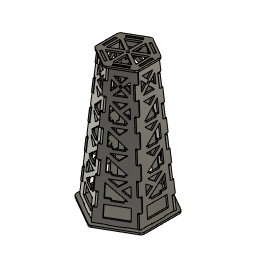
windmill v4 (Autodesk Fusion 360 design; units mm, degrees)
Autodesk Fusion 360 part; units mm, degrees
sketch "Sketch2" plane through (0, 0, 0) normal (0, 0, 1) x (1, 0, 0)
  line L0 (129.0294, -114.8559) -> (68.6327, -149.726)
  arc A0 (68.6327, -149.726) -> (63.1421, -149.726) centre (65.8874, -144.9709) cw
  line L1 (63.1421, -149.726) -> (2.7453, -114.8559)
  arc A1 (2.7453, -114.8559) -> (0, -110.1009) centre (5.4906, -110.1009) cw
  line L2 (0, -110.1009) -> (0, -40.3607)
  arc A2 (0, -40.3607) -> (2.7453, -35.6057) centre (5.4906, -40.3607) cw
  line L3 (2.7453, -35.6057) -> (63.1421, -0.7356)
  arc A3 (63.1421, -0.7356) -> (68.6327, -0.7356) centre (65.8874, -5.4906) cw
  line L4 (68.6327, -0.7356) -> (129.0294, -35.6057)
  arc A4 (129.0294, -35.6057) -> (131.7748, -40.3607) centre (126.2841, -40.3607) cw
  line L5 (131.7748, -40.3607) -> (131.7748, -110.1009)
  arc A5 (131.7748, -110.1009) -> (129.0294, -114.8559) centre (126.2841, -110.1009) cw
  line L6 (84.6564, -133.0999) -> (106.6189, -120.4198)
  line L7 (106.6189, -120.4198) -> (104.7697, -117.217)
  line L8 (104.7697, -117.217) -> (82.8073, -129.897)
  line L9 (82.8073, -129.897) -> (84.6564, -133.0999)
  line L10 (47.1183, -133.0997) -> (25.1558, -120.4197)
  line L11 (25.1558, -120.4197) -> (27.005, -117.2168)
  line L12 (27.005, -117.2168) -> (48.9674, -129.8969)
  line L13 (48.9674, -129.8969) -> (47.1183, -133.0997)
  line L14 (47.1183, -17.3616) -> (25.1558, -30.0416)
  line L15 (25.1558, -30.0416) -> (27.005, -33.2445)
  line L16 (27.005, -33.2445) -> (48.9674, -20.5645)
  line L17 (48.9674, -20.5645) -> (47.1183, -17.3616)
  line L18 (121.6896, -62.5506) -> (125.388, -62.5506)
  line L19 (125.388, -62.5506) -> (125.388, -87.9107)
  line L20 (125.388, -87.9107) -> (121.6896, -87.9107)
  line L21 (121.6896, -87.9107) -> (121.6896, -62.5506)
  line L22 (6.3867, -62.5506) -> (10.0851, -62.5506)
  line L23 (10.0851, -62.5506) -> (10.0851, -87.9107)
  line L24 (10.0851, -87.9107) -> (6.3867, -87.9107)
  line L25 (6.3867, -87.9107) -> (6.3867, -62.5506)
  line L26 (84.6564, -17.3616) -> (106.6189, -30.0416)
  line L27 (106.6189, -30.0416) -> (104.7697, -33.2445)
  line L28 (104.7697, -33.2445) -> (82.8073, -20.5645)
  line L29 (82.8073, -20.5645) -> (84.6564, -17.3616)
extrude "Extrude1" add sketch "Sketch2" along normal blind 3.175 makes body 1
sketch "Sketch4" plane through (0, 0, 0) normal (0, 0, 1) x (1, 0, 0)
  line L0 (18.968, -3.1158) -> (17.7262, -25.4072)
  line L1 (17.7262, -25.4072) -> (11.8611, -25.4072)
  arc A0 (11.3622, -25.8815) -> (11.8611, -25.4072) centre (11.8611, -25.9067) cw
  line L2 (11.3622, -25.8815) -> (10.145, -49.9595)
  arc A1 (10.6433, -50.4837) -> (10.145, -49.9595) centre (10.6433, -49.9847) cw
  line L3 (10.6433, -50.4837) -> (16.4585, -50.4837)
  line L4 (16.4585, -50.4837) -> (15.1903, -76.1274)
  line L5 (15.1903, -76.1274) -> (9.3252, -76.1274)
  arc A2 (8.8263, -76.6016) -> (9.3252, -76.1274) centre (9.3252, -76.6269) cw
  line L6 (8.8263, -76.6016) -> (7.6091, -100.6797)
  arc A3 (8.1074, -101.2038) -> (7.6091, -100.6797) centre (8.1074, -100.7049) cw
  line L7 (8.1074, -101.2038) -> (13.9226, -101.2038)
  line L8 (13.9226, -101.2038) -> (12.6544, -126.8475)
  line L9 (12.6544, -126.8475) -> (6.7893, -126.8475)
  arc A4 (6.2904, -127.3218) -> (6.7893, -126.8475) centre (6.7893, -127.347) cw
  line L10 (6.2904, -127.3218) -> (5.0727, -151.3998)
  arc A5 (5.571, -151.9239) -> (5.0727, -151.3998) centre (5.571, -151.425) cw
  line L11 (5.571, -151.9239) -> (11.3862, -151.9239)
  line L12 (11.3862, -151.9239) -> (10.1185, -177.5676)
  line L13 (10.1185, -177.5676) -> (4.2534, -177.5676)
  arc A6 (3.7545, -178.0419) -> (4.2534, -177.5676) centre (4.2534, -178.0671) cw
  line L14 (3.7545, -178.0419) -> (2.5368, -202.1199)
  arc A7 (3.0351, -202.644) -> (2.5368, -202.1199) centre (3.0351, -202.1451) cw
  line L15 (3.0351, -202.644) -> (8.8503, -202.644)
  line L16 (8.8503, -202.644) -> (7.5826, -228.2878)
  line L17 (7.5826, -228.2878) -> (1.7174, -228.2878)
  arc A8 (1.2188, -228.762) -> (1.7174, -228.2878) centre (1.7174, -228.787) cw
  line L18 (1.2188, -228.762) -> (0.0006, -253.0765)
  arc A9 (0.4992, -253.6006) -> (0.0006, -253.0765) centre (0.4992, -253.1015) cw
  line L19 (0.4992, -253.6006) -> (23.7494, -253.6006)
  line L20 (23.7494, -253.6006) -> (23.7494, -255.7351)
  arc A10 (24.2566, -256.2423) -> (23.7494, -255.7351) centre (24.2566, -255.7351) cw
  line L21 (24.2566, -256.2423) -> (48.6023, -256.2423)
  arc A11 (49.1095, -255.7351) -> (48.6023, -256.2423) centre (48.6023, -255.7351) cw
  line L22 (49.1095, -255.7351) -> (49.1095, -253.6006)
  line L23 (49.1095, -253.6006) -> (66.0203, -253.6006)
  arc A12 (66.5186, -253.077) -> (66.0203, -253.6006) centre (66.0203, -253.1017) cw
  line L24 (66.5186, -253.077) -> (65.2763, -228.0041)
  line L25 (65.2763, -228.0041) -> (71.0904, -228.0041)
  arc A13 (71.5898, -227.4788) -> (71.0904, -228.0041) centre (71.0904, -227.5041) cw
  line L26 (71.5898, -227.4788) -> (70.3726, -203.4009)
  arc A14 (69.8748, -202.9277) -> (70.3726, -203.4009) centre (69.8748, -203.4261) cw
  line L27 (69.8748, -202.9277) -> (64.0086, -202.9277)
  line L28 (64.0086, -202.9277) -> (62.7404, -177.284)
  line L29 (62.7404, -177.284) -> (68.5545, -177.284)
  arc A15 (69.0539, -176.7587) -> (68.5545, -177.284) centre (68.5545, -176.784) cw
  line L30 (69.0539, -176.7587) -> (67.8367, -152.6808)
  arc A16 (67.3389, -152.2076) -> (67.8367, -152.6808) centre (67.3389, -152.706) cw
  line L31 (67.3389, -152.2076) -> (61.4727, -152.2076)
  line L32 (61.4727, -152.2076) -> (60.2058, -126.5889)
  arc A17 (60.2058, -126.5889) -> (60.2296, -126.5639) centre (60.2296, -126.5878) cw
  line L33 (60.2296, -126.5639) -> (66.0186, -126.5639)
  arc A18 (66.518, -126.0386) -> (66.0186, -126.5639) centre (66.0186, -126.0639) cw
  line L34 (66.518, -126.0386) -> (65.3016, -101.9861)
  arc A19 (64.7771, -101.4875) -> (65.3016, -101.9861) centre (64.7771, -102.0126) cw
  line L35 (64.7771, -101.4875) -> (58.9363, -101.4875)
  line L36 (58.9363, -101.4875) -> (57.6686, -75.8438)
  line L37 (57.6686, -75.8438) -> (63.4827, -75.8438)
  arc A20 (63.9821, -75.3184) -> (63.4827, -75.8438) centre (63.4827, -75.3437) cw
  line L38 (63.9821, -75.3184) -> (62.7643, -51.2405)
  arc A21 (62.2666, -50.7673) -> (62.7643, -51.2405) centre (62.2666, -51.2657) cw
  line L39 (62.2666, -50.7673) -> (56.4004, -50.7673)
  line L40 (56.4004, -50.7673) -> (55.1327, -25.1236)
  line L41 (55.1327, -25.1236) -> (60.9474, -25.1236)
  arc A22 (61.4431, -24.5991) -> (60.9474, -25.1236) centre (60.9474, -24.627) cw
  line L42 (61.4431, -24.5991) -> (60.2312, -3.1153)
  arc A23 (59.7301, -2.6417) -> (60.2312, -3.1153) centre (59.7301, -3.1436) cw
  line L43 (59.7301, -2.6417) -> (49.1095, -2.6417)
  line L44 (49.1095, -2.6417) -> (49.1095, -0.5072)
  arc A24 (48.6023, 0) -> (49.1095, -0.5072) centre (48.6023, -0.5072) cw
  line L45 (48.6023, 0) -> (24.2566, 0)
  arc A25 (23.7494, -0.5072) -> (24.2566, 0) centre (24.2566, -0.5072) cw
  line L46 (23.7494, -0.5072) -> (23.7494, -2.6417)
  line L47 (23.7494, -2.6417) -> (19.4693, -2.6417)
  arc A26 (18.968, -3.1158) -> (19.4693, -2.6417) centre (19.4693, -3.1437) cw
  line L48 (21.7542, -63.9071) -> (20.9934, -88.2533)
  arc A27 (21.4847, -88.7602) -> (20.9934, -88.2533) centre (21.4847, -88.2686) cw
  line L49 (21.4847, -88.7602) -> (26.412, -88.7602)
  arc A28 (26.412, -88.7602) -> (26.9192, -89.2674) centre (26.412, -89.2674) cw
  line L50 (26.9192, -89.2674) -> (26.9192, -91.9302)
  line L51 (26.9192, -91.9302) -> (45.9393, -91.9302)
  line L52 (45.9393, -91.9302) -> (45.9393, -89.2674)
  arc A29 (45.9393, -89.2674) -> (46.4465, -88.7602) centre (46.4465, -89.2674) cw
  line L53 (46.4465, -88.7602) -> (47.8116, -88.7602)
  arc A30 (47.9521, -88.4099) -> (47.8116, -88.7602) centre (47.8116, -88.5569) cw
  line L54 (47.9521, -88.4099) -> (22.1368, -63.7505)
  arc A31 (21.7542, -63.9071) -> (22.1368, -63.7505) centre (21.9804, -63.9142) cw
  line L55 (20.4659, -105.1172) -> (19.705, -129.4634)
  arc A32 (20.1964, -129.9703) -> (19.705, -129.4634) centre (20.1964, -129.4787) cw
  line L56 (20.1964, -129.9703) -> (26.412, -129.9703)
  arc A33 (26.412, -129.9703) -> (26.9192, -130.4775) centre (26.412, -130.4775) cw
  line L57 (26.9192, -130.4775) -> (26.9192, -133.1403)
  line L58 (26.9192, -133.1403) -> (45.9393, -133.1403)
  line L59 (45.9393, -133.1403) -> (45.9393, -130.4775)
  arc A34 (45.9393, -130.4775) -> (46.4465, -129.9703) centre (46.4465, -130.4775) cw
  line L60 (46.4465, -129.9703) -> (48.8017, -129.9703)
  arc A35 (48.9281, -129.6353) -> (48.8017, -129.9703) centre (48.8018, -129.779) cw
  line L61 (48.9281, -129.6353) -> (20.8625, -104.9453)
  arc A36 (20.4659, -105.1172) -> (20.8625, -104.9453) centre (20.7047, -105.1247) cw
  line L62 (19.1775, -146.3273) -> (18.4167, -170.6735)
  arc A37 (18.9081, -171.1804) -> (18.4167, -170.6735) centre (18.9081, -170.6888) cw
  line L63 (18.9081, -171.1804) -> (26.412, -171.1804)
  arc A38 (26.412, -171.1804) -> (26.9192, -171.6876) centre (26.412, -171.6876) cw
  line L64 (26.9192, -171.6876) -> (26.9192, -174.3504)
  line L65 (26.9192, -174.3504) -> (45.9393, -174.3504)
  line L66 (45.9393, -174.3504) -> (45.9393, -171.6876)
  arc A39 (45.9393, -171.6876) -> (46.4465, -171.1804) centre (46.4465, -171.6876) cw
  line L67 (46.4465, -171.1804) -> (49.7919, -171.1804)
  arc A40 (49.906, -170.8599) -> (49.7919, -171.1804) centre (49.7919, -170.9999) cw
  line L68 (49.906, -170.8599) -> (19.5865, -146.1409)
  arc A41 (19.1775, -146.3273) -> (19.5865, -146.1409) centre (19.4281, -146.3351) cw
  line L69 (17.8897, -187.5374) -> (17.1284, -211.8836)
  arc A42 (17.6197, -212.3905) -> (17.1284, -211.8836) centre (17.6197, -211.8989) cw
  line L70 (17.6197, -212.3905) -> (26.412, -212.3905)
  arc A43 (26.412, -212.3905) -> (26.9192, -212.8977) centre (26.412, -212.8977) cw
  line L71 (26.9192, -212.8977) -> (26.9192, -215.5605)
  line L72 (26.9192, -215.5605) -> (45.9393, -215.5605)
  line L73 (45.9393, -215.5605) -> (45.9393, -212.8977)
  arc A44 (45.9393, -212.8977) -> (46.4465, -212.3905) centre (46.4465, -212.8977) cw
  line L74 (46.4465, -212.3905) -> (50.782, -212.3905)
  arc A45 (50.8853, -212.0837) -> (50.782, -212.3905) centre (50.782, -212.2197) cw
  line L75 (50.8853, -212.0837) -> (18.3094, -187.3373)
  arc A46 (17.8897, -187.5374) -> (18.3094, -187.3373) centre (18.1512, -187.5456) cw
  line L76 (54.5485, -187.334) -> (42.6278, -196.237)
  arc A47 (42.6342, -196.8351) -> (42.6278, -196.237) centre (42.8493, -196.5337) cw
  line L77 (42.6342, -196.8351) -> (55.1362, -205.7559)
  arc A48 (55.5332, -205.5436) -> (55.1362, -205.7559) centre (55.2821, -205.5514) cw
  line L78 (55.5332, -205.5436) -> (54.9707, -187.5374)
  arc A49 (54.5485, -187.334) -> (54.9707, -187.5374) centre (54.7066, -187.5457) cw
  line L79 (22.84, -180.6905) -> (50.0204, -180.6905)
  arc A50 (50.0204, -180.6905) -> (50.129, -181.0041) centre (50.0204, -180.8661) cw
  line L80 (50.129, -181.0041) -> (36.8286, -191.4718)
  arc A51 (36.8286, -191.4718) -> (36.0315, -191.4718) centre (36.4301, -190.9654) cw
  line L81 (36.0315, -191.4718) -> (22.7313, -181.0041)
  arc A52 (22.7313, -181.0041) -> (22.84, -180.6905) centre (22.84, -180.8661) cw
  line L82 (53.272, -146.138) -> (42.221, -155.0128)
  arc A53 (42.2284, -155.6385) -> (42.221, -155.0128) centre (42.4699, -155.3228) cw
  line L83 (42.2284, -155.6385) -> (53.8587, -164.5323)
  arc A54 (54.2457, -164.3335) -> (53.8587, -164.5323) centre (54.005, -164.341) cw
  line L84 (54.2457, -164.3335) -> (53.6832, -146.3273)
  arc A55 (53.2719, -146.138) -> (53.6832, -146.3273) centre (53.4303, -146.3352) cw
  line L85 (23.831, -139.4803) -> (49.0301, -139.4803)
  arc A56 (49.0301, -139.4803) -> (49.1502, -139.808) centre (49.0301, -139.6662) cw
  line L86 (49.1502, -139.808) -> (36.8176, -150.2477)
  arc A57 (36.8176, -150.2477) -> (36.0433, -150.2477) centre (36.4305, -149.7903) cw
  line L87 (36.0433, -150.2477) -> (23.7109, -139.808)
  arc A58 (23.7109, -139.808) -> (23.831, -139.4803) centre (23.831, -139.6662) cw
  line L88 (51.9971, -104.9428) -> (41.8126, -113.7877)
  arc A59 (41.8211, -114.4428) -> (41.8126, -113.7877) centre (42.0939, -114.1116) cw
  line L89 (41.8211, -114.4428) -> (52.5827, -123.3078)
  arc A60 (52.9583, -123.1233) -> (52.5827, -123.3078) centre (52.7287, -123.1305) cw
  line L90 (52.9583, -123.1233) -> (52.3958, -105.1172)
  arc A61 (51.9971, -104.9428) -> (52.3958, -105.1172) centre (52.155, -105.1247) cw
  line L91 (24.8221, -98.2702) -> (48.0399, -98.2702)
  arc A62 (48.0399, -98.2702) -> (48.1731, -98.6128) centre (48.0399, -98.4674) cw
  line L92 (48.1731, -98.6128) -> (36.8049, -109.0227)
  arc A63 (36.8049, -109.0227) -> (36.0568, -109.0227) centre (36.4309, -108.6142) cw
  line L93 (36.0568, -109.0227) -> (24.6889, -98.6128)
  arc A64 (24.6889, -98.6128) -> (24.8221, -98.2702) centre (24.822, -98.4674) cw
  line L94 (50.7241, -63.7486) -> (41.4024, -72.5617)
  arc A65 (41.4122, -73.248) -> (41.4024, -72.5617) centre (41.7225, -72.9003) cw
  line L95 (41.4122, -73.248) -> (51.3084, -82.0824)
  arc A66 (51.6709, -81.9132) -> (51.3084, -82.0824) centre (51.4534, -81.92) cw
  line L96 (51.6709, -81.9132) -> (51.1084, -63.9071)
  arc A67 (50.7241, -63.7486) -> (51.1084, -63.9071) centre (50.8806, -63.9142) cw
  line L97 (25.8131, -57.0601) -> (47.0497, -57.0601)
  arc A68 (47.0497, -57.0601) -> (47.1978, -57.4183) centre (47.0497, -57.2698) cw
  line L98 (47.1978, -57.4183) -> (36.7904, -67.797)
  arc A69 (36.7904, -67.797) -> (36.0721, -67.797) centre (36.4313, -67.4369) cw
  line L99 (36.0721, -67.797) -> (25.665, -57.4183)
  arc A70 (25.665, -57.4183) -> (25.8131, -57.0601) centre (25.8131, -57.2698) cw
  line L100 (49.4532, -22.5552) -> (40.99, -31.3349)
  arc A71 (41.0013, -32.054) -> (40.99, -31.3349) centre (41.3571, -31.6888) cw
  line L101 (41.0013, -32.054) -> (50.0361, -40.8562)
  arc A72 (50.3836, -40.7032) -> (50.0361, -40.8562) centre (50.179, -40.7095) cw
  line L102 (50.3836, -40.7032) -> (49.821, -22.697)
  arc A73 (49.4532, -22.5552) -> (49.821, -22.697) centre (49.6072, -22.7037) cw
  line L103 (23.4103, -22.5552) -> (31.8733, -31.3349)
  arc A74 (31.8733, -31.3349) -> (31.862, -32.054) centre (31.5062, -31.6888) cw
  line L104 (31.862, -32.054) -> (22.827, -40.8562)
  arc A75 (22.827, -40.8562) -> (22.4795, -40.7032) centre (22.6842, -40.7095) cw
  line L105 (22.4795, -40.7032) -> (23.0424, -22.697)
  arc A76 (23.0424, -22.697) -> (23.4103, -22.5552) centre (23.2562, -22.7037) cw
  line L106 (26.0418, -47.5501) -> (46.8212, -47.5501)
  arc A77 (46.973, -47.1883) -> (46.8212, -47.5501) centre (46.8212, -47.3373) cw
  line L107 (46.973, -47.1883) -> (36.787, -36.817)
  arc A78 (36.0762, -36.8169) -> (36.787, -36.817) centre (36.4316, -37.166) cw
  line L108 (36.0762, -36.8169) -> (25.89, -47.1883)
  arc A79 (26.0418, -47.5501) -> (25.89, -47.1883) centre (26.0418, -47.3373) cw
  line L109 (26.8041, -15.85) -> (46.0595, -15.85)
  arc A80 (46.0595, -15.85) -> (46.2246, -16.2245) centre (46.0595, -16.0737) cw
  line L110 (46.2246, -16.2245) -> (36.7738, -26.5706)
  arc A81 (36.7738, -26.5706) -> (36.0896, -26.5706) centre (36.4317, -26.2581) cw
  line L111 (36.0896, -26.5706) -> (26.639, -16.2245)
  arc A82 (26.639, -16.2245) -> (26.8041, -15.85) centre (26.8041, -16.0737) cw
  line L112 (56.7216, -243.5837) -> (56.06, -222.4075)
  arc A83 (55.537, -221.9006) -> (56.06, -222.4075) centre (55.537, -222.4238) cw
  line L113 (55.537, -221.9006) -> (17.3225, -221.9006)
  arc A84 (16.7995, -222.4075) -> (17.3225, -221.9006) centre (17.3225, -222.4239) cw
  line L114 (16.7995, -222.4075) -> (16.1375, -243.5837)
  arc A85 (16.6289, -244.0906) -> (16.1375, -243.5837) centre (16.6289, -243.599) cw
  line L115 (16.6289, -244.0906) -> (56.2302, -244.0906)
  arc A86 (56.7216, -243.5837) -> (56.2302, -244.0906) centre (56.2302, -243.599) cw
  spline S0 degree 3 poles (36.4311, -34.1415) (35.0825, -34.1417) (33.989, -33.0487) (33.9885, -31.7001) knots 0 0 0 0 1 1 1 1
  spline S1 degree 3 poles (33.9885, -31.7001) (33.988, -30.3515) (35.0808, -29.2578) (36.4294, -29.2571) knots 0 0 0 0 1 1 1 1
  spline S2 degree 3 poles (36.4294, -29.2571) (37.778, -29.2564) (38.8719, -30.349) (38.8724, -31.6984) knots 0 0 0 0 1 1 1 1
  spline S3 degree 3 poles (38.8724, -31.6984) (38.8728, -33.0479) (37.7797, -34.1412) (36.4311, -34.1415) knots 0 0 0 0 1 1 1 1
move_body "Move1" bodies 1 to x (1, 0, 0) y (0, 1, 0) z (0, 0, 1) at (101.6, 0, 0)
extrude "Extrude2" add sketch "Sketch4" along normal blind 3.175 separate body contours L0 L1 A0 L2 A1 L3 L4 L5 A2 L6 A3 L7 L8 L9 A4 L10 A5 L11 L12 L13 A6 L14 A7 L15 L16 L17 A8 L18 A9 L19 L20 A10 L21 A11 L22 L23 A12 L24 L25 A13 L26 A14 L27 L28 L29 A15 L30 A16 L31 L32 A17 L33 A18 L34 A19 L35 L36 L37 A20 L38 A21 L39 L40 L41 A22 L42 A23 L43 L44 A24 L45 A25 L46 L47 A26 | L82 A53 L83 A54 L84 A55 | L88 A59 L89 A60 L90 A61 makes body 2
move_body "Move2" bodies 2 to x (1, 0, 0) y (0, 1, 0) z (0, 0, 1) at (241.3, 0, 0)
sketch "Sketch5" plane through (0, 0, 0) normal (0, 0, 1) x (1, 0, 0)
  line L0 (18.968, -3.1158) -> (17.7262, -25.4072)
  line L1 (17.7262, -25.4072) -> (11.8611, -25.4072)
  arc A0 (11.3622, -25.8815) -> (11.8611, -25.4072) centre (11.8611, -25.9067) cw
  line L2 (11.3622, -25.8815) -> (10.145, -49.9595)
  arc A1 (10.6433, -50.4837) -> (10.145, -49.9595) centre (10.6433, -49.9847) cw
  line L3 (10.6433, -50.4837) -> (16.4585, -50.4837)
  line L4 (16.4585, -50.4837) -> (15.1903, -76.1274)
  line L5 (15.1903, -76.1274) -> (9.3252, -76.1274)
  arc A2 (8.8263, -76.6016) -> (9.3252, -76.1274) centre (9.3252, -76.6269) cw
  line L6 (8.8263, -76.6016) -> (7.6091, -100.6797)
  arc A3 (8.1074, -101.2038) -> (7.6091, -100.6797) centre (8.1074, -100.7049) cw
  line L7 (8.1074, -101.2038) -> (13.9226, -101.2038)
  line L8 (13.9226, -101.2038) -> (12.6544, -126.8475)
  line L9 (12.6544, -126.8475) -> (6.7893, -126.8475)
  arc A4 (6.2904, -127.3218) -> (6.7893, -126.8475) centre (6.7893, -127.347) cw
  line L10 (6.2904, -127.3218) -> (5.0727, -151.3998)
  arc A5 (5.571, -151.9239) -> (5.0727, -151.3998) centre (5.571, -151.425) cw
  line L11 (5.571, -151.9239) -> (11.3862, -151.9239)
  line L12 (11.3862, -151.9239) -> (10.1185, -177.5676)
  line L13 (10.1185, -177.5676) -> (4.2534, -177.5676)
  arc A6 (3.7545, -178.0419) -> (4.2534, -177.5676) centre (4.2534, -178.0671) cw
  line L14 (3.7545, -178.0419) -> (2.5368, -202.1199)
  arc A7 (3.0351, -202.644) -> (2.5368, -202.1199) centre (3.0351, -202.1451) cw
  line L15 (3.0351, -202.644) -> (8.8503, -202.644)
  line L16 (8.8503, -202.644) -> (7.5826, -228.2878)
  line L17 (7.5826, -228.2878) -> (1.7174, -228.2878)
  arc A8 (1.2188, -228.762) -> (1.7174, -228.2878) centre (1.7174, -228.787) cw
  line L18 (1.2188, -228.762) -> (0.0006, -253.0765)
  arc A9 (0.4992, -253.6006) -> (0.0006, -253.0765) centre (0.4992, -253.1015) cw
  line L19 (0.4992, -253.6006) -> (23.7494, -253.6006)
  line L20 (23.7494, -253.6006) -> (23.7494, -255.7351)
  arc A10 (24.2566, -256.2423) -> (23.7494, -255.7351) centre (24.2566, -255.7351) cw
  line L21 (24.2566, -256.2423) -> (48.6023, -256.2423)
  arc A11 (49.1095, -255.7351) -> (48.6023, -256.2423) centre (48.6023, -255.7351) cw
  line L22 (49.1095, -255.7351) -> (49.1095, -253.6006)
  line L23 (49.1095, -253.6006) -> (66.0203, -253.6006)
  arc A12 (66.5186, -253.077) -> (66.0203, -253.6006) centre (66.0203, -253.1017) cw
  line L24 (66.5186, -253.077) -> (65.2763, -228.0041)
  line L25 (65.2763, -228.0041) -> (71.0904, -228.0041)
  arc A13 (71.5898, -227.4788) -> (71.0904, -228.0041) centre (71.0904, -227.5041) cw
  line L26 (71.5898, -227.4788) -> (70.3726, -203.4009)
  arc A14 (69.8748, -202.9277) -> (70.3726, -203.4009) centre (69.8748, -203.4261) cw
  line L27 (69.8748, -202.9277) -> (64.0086, -202.9277)
  line L28 (64.0086, -202.9277) -> (62.7404, -177.284)
  line L29 (62.7404, -177.284) -> (68.5545, -177.284)
  arc A15 (69.0539, -176.7587) -> (68.5545, -177.284) centre (68.5545, -176.784) cw
  line L30 (69.0539, -176.7587) -> (67.8367, -152.6808)
  arc A16 (67.3389, -152.2076) -> (67.8367, -152.6808) centre (67.3389, -152.706) cw
  line L31 (67.3389, -152.2076) -> (61.4727, -152.2076)
  line L32 (61.4727, -152.2076) -> (60.2058, -126.5889)
  arc A17 (60.2058, -126.5889) -> (60.2296, -126.5639) centre (60.2296, -126.5878) cw
  line L33 (60.2296, -126.5639) -> (66.0186, -126.5639)
  arc A18 (66.518, -126.0386) -> (66.0186, -126.5639) centre (66.0186, -126.0639) cw
  line L34 (66.518, -126.0386) -> (65.3016, -101.9861)
  arc A19 (64.7771, -101.4875) -> (65.3016, -101.9861) centre (64.7771, -102.0126) cw
  line L35 (64.7771, -101.4875) -> (58.9363, -101.4875)
  line L36 (58.9363, -101.4875) -> (57.6686, -75.8438)
  line L37 (57.6686, -75.8438) -> (63.4827, -75.8438)
  arc A20 (63.9821, -75.3184) -> (63.4827, -75.8438) centre (63.4827, -75.3437) cw
  line L38 (63.9821, -75.3184) -> (62.7643, -51.2405)
  arc A21 (62.2666, -50.7673) -> (62.7643, -51.2405) centre (62.2666, -51.2657) cw
  line L39 (62.2666, -50.7673) -> (56.4004, -50.7673)
  line L40 (56.4004, -50.7673) -> (55.1327, -25.1236)
  line L41 (55.1327, -25.1236) -> (60.9474, -25.1236)
  arc A22 (61.4431, -24.5991) -> (60.9474, -25.1236) centre (60.9474, -24.627) cw
  line L42 (61.4431, -24.5991) -> (60.2312, -3.1153)
  arc A23 (59.7301, -2.6417) -> (60.2312, -3.1153) centre (59.7301, -3.1436) cw
  line L43 (59.7301, -2.6417) -> (49.1095, -2.6417)
  line L44 (49.1095, -2.6417) -> (49.1095, -0.5072)
  arc A24 (48.6023, 0) -> (49.1095, -0.5072) centre (48.6023, -0.5072) cw
  line L45 (48.6023, 0) -> (24.2566, 0)
  arc A25 (23.7494, -0.5072) -> (24.2566, 0) centre (24.2566, -0.5072) cw
  line L46 (23.7494, -0.5072) -> (23.7494, -2.6417)
  line L47 (23.7494, -2.6417) -> (19.4693, -2.6417)
  arc A26 (18.968, -3.1158) -> (19.4693, -2.6417) centre (19.4693, -3.1437) cw
  line L48 (51.1053, -63.9071) -> (51.8662, -88.2533)
  arc A27 (51.8662, -88.2533) -> (51.3748, -88.7602) centre (51.3748, -88.2686) cw
  line L49 (51.3748, -88.7602) -> (46.4475, -88.7602)
  arc A28 (45.9403, -89.2674) -> (46.4475, -88.7602) centre (46.4475, -89.2674) cw
  line L50 (45.9403, -89.2674) -> (45.9403, -91.9302)
  line L51 (45.9403, -91.9302) -> (26.9202, -91.9302)
  line L52 (26.9202, -91.9302) -> (26.9202, -89.2674)
  arc A29 (26.413, -88.7602) -> (26.9202, -89.2674) centre (26.413, -89.2674) cw
  line L53 (26.413, -88.7602) -> (25.0479, -88.7602)
  arc A30 (25.0479, -88.7602) -> (24.9074, -88.4099) centre (25.0479, -88.5569) cw
  line L54 (24.9074, -88.4099) -> (50.7227, -63.7505)
  arc A31 (50.7227, -63.7505) -> (51.1053, -63.9071) centre (50.8791, -63.9142) cw
  line L55 (52.3937, -105.1172) -> (53.1545, -129.4634)
  arc A32 (53.1545, -129.4634) -> (52.6631, -129.9703) centre (52.6631, -129.4787) cw
  line L56 (52.6631, -129.9703) -> (46.4475, -129.9703)
  arc A33 (45.9403, -130.4775) -> (46.4475, -129.9703) centre (46.4475, -130.4775) cw
  line L57 (45.9403, -130.4775) -> (45.9403, -133.1403)
  line L58 (45.9403, -133.1403) -> (26.9202, -133.1403)
  line L59 (26.9202, -133.1403) -> (26.9202, -130.4775)
  arc A34 (26.413, -129.9703) -> (26.9202, -130.4775) centre (26.413, -130.4775) cw
  line L60 (26.413, -129.9703) -> (24.0578, -129.9703)
  arc A35 (24.0578, -129.9703) -> (23.9314, -129.6353) centre (24.0578, -129.779) cw
  line L61 (23.9314, -129.6353) -> (51.997, -104.9453)
  arc A36 (51.997, -104.9453) -> (52.3937, -105.1172) centre (52.1548, -105.1247) cw
  line L62 (53.682, -146.3273) -> (54.4428, -170.6735)
  arc A37 (54.4428, -170.6735) -> (53.9515, -171.1804) centre (53.9515, -170.6888) cw
  line L63 (53.9515, -171.1804) -> (46.4475, -171.1804)
  arc A38 (45.9403, -171.6876) -> (46.4475, -171.1804) centre (46.4475, -171.6876) cw
  line L64 (45.9403, -171.6876) -> (45.9403, -174.3504)
  line L65 (45.9403, -174.3504) -> (26.9202, -174.3504)
  line L66 (26.9202, -174.3504) -> (26.9202, -171.6876)
  arc A39 (26.413, -171.1804) -> (26.9202, -171.6876) centre (26.413, -171.6876) cw
  line L67 (26.413, -171.1804) -> (23.0677, -171.1804)
  arc A40 (23.0677, -171.1804) -> (22.9536, -170.8599) centre (23.0677, -170.9999) cw
  line L68 (22.9536, -170.8599) -> (53.2731, -146.1409)
  arc A41 (53.2731, -146.1409) -> (53.682, -146.3273) centre (53.4315, -146.3351) cw
  line L69 (54.9698, -187.5374) -> (55.7311, -211.8836)
  arc A42 (55.7311, -211.8836) -> (55.2398, -212.3905) centre (55.2398, -211.8989) cw
  line L70 (55.2398, -212.3905) -> (46.4475, -212.3905)
  arc A43 (45.9403, -212.8977) -> (46.4475, -212.3905) centre (46.4475, -212.8977) cw
  line L71 (45.9403, -212.8977) -> (45.9403, -215.5605)
  line L72 (45.9403, -215.5605) -> (26.9202, -215.5605)
  line L73 (26.9202, -215.5605) -> (26.9202, -212.8977)
  arc A44 (26.413, -212.3905) -> (26.9202, -212.8977) centre (26.413, -212.8977) cw
  line L74 (26.413, -212.3905) -> (22.0775, -212.3905)
  arc A45 (22.0775, -212.3905) -> (21.9742, -212.0837) centre (22.0775, -212.2197) cw
  line L75 (21.9742, -212.0837) -> (54.5501, -187.3373)
  arc A46 (54.5501, -187.3373) -> (54.9698, -187.5374) centre (54.7083, -187.5456) cw
  line L76 (18.311, -187.334) -> (30.2318, -196.237)
  arc A47 (30.2318, -196.237) -> (30.2253, -196.8351) centre (30.0102, -196.5337) cw
  line L77 (30.2253, -196.8351) -> (17.7234, -205.7559)
  arc A48 (17.7234, -205.7559) -> (17.3263, -205.5436) centre (17.5774, -205.5514) cw
  line L78 (17.3263, -205.5436) -> (17.8888, -187.5374)
  arc A49 (17.8888, -187.5374) -> (18.3111, -187.334) centre (18.1529, -187.5457) cw
  line L79 (50.0195, -180.6905) -> (22.8392, -180.6905)
  arc A50 (22.7305, -181.0041) -> (22.8392, -180.6905) centre (22.8392, -180.8661) cw
  line L80 (22.7305, -181.0041) -> (36.0309, -191.4718)
  arc A51 (36.828, -191.4718) -> (36.0309, -191.4718) centre (36.4295, -190.9654) cw
  line L81 (36.828, -191.4718) -> (50.1282, -181.0041)
  arc A52 (50.0195, -180.6905) -> (50.1282, -181.0041) centre (50.0195, -180.8661) cw
  line L82 (19.5875, -146.138) -> (30.6385, -155.0128)
  arc A53 (30.6385, -155.0128) -> (30.6311, -155.6385) centre (30.3897, -155.3228) cw
  line L83 (30.6311, -155.6385) -> (19.0008, -164.5323)
  arc A54 (19.0008, -164.5323) -> (18.6138, -164.3335) centre (18.8545, -164.341) cw
  line L84 (18.6138, -164.3335) -> (19.1763, -146.3273)
  arc A55 (19.1763, -146.3273) -> (19.5876, -146.138) centre (19.4292, -146.3352) cw
  line L85 (49.0285, -139.4803) -> (23.8294, -139.4803)
  arc A56 (23.7093, -139.808) -> (23.8294, -139.4803) centre (23.8294, -139.6662) cw
  line L86 (23.7093, -139.808) -> (36.0419, -150.2477)
  arc A57 (36.8162, -150.2477) -> (36.0419, -150.2477) centre (36.429, -149.7903) cw
  line L87 (36.8162, -150.2477) -> (49.1486, -139.808)
  arc A58 (49.0285, -139.4803) -> (49.1486, -139.808) centre (49.0285, -139.6662) cw
  line L88 (20.8624, -104.9428) -> (31.0469, -113.7877)
  arc A59 (31.0469, -113.7877) -> (31.0384, -114.4428) centre (30.7656, -114.1116) cw
  line L89 (31.0384, -114.4428) -> (20.2768, -123.3078)
  arc A60 (20.2768, -123.3078) -> (19.9012, -123.1233) centre (20.1308, -123.1305) cw
  line L90 (19.9012, -123.1233) -> (20.4637, -105.1172)
  arc A61 (20.4637, -105.1172) -> (20.8625, -104.9428) centre (20.7045, -105.1247) cw
  line L91 (48.0375, -98.2702) -> (24.8196, -98.2702)
  arc A62 (24.6865, -98.6128) -> (24.8196, -98.2702) centre (24.8196, -98.4674) cw
  line L92 (24.6865, -98.6128) -> (36.0546, -109.0227)
  arc A63 (36.8027, -109.0227) -> (36.0546, -109.0227) centre (36.4286, -108.6142) cw
  line L93 (36.8027, -109.0227) -> (48.1706, -98.6128)
  arc A64 (48.0375, -98.2702) -> (48.1706, -98.6128) centre (48.0375, -98.4674) cw
  line L94 (22.1355, -63.7486) -> (31.4571, -72.5617)
  arc A65 (31.4571, -72.5617) -> (31.4473, -73.248) centre (31.137, -72.9003) cw
  line L95 (31.4473, -73.248) -> (21.5511, -82.0824)
  arc A66 (21.5511, -82.0824) -> (21.1886, -81.9132) centre (21.4061, -81.92) cw
  line L96 (21.1886, -81.9132) -> (21.7511, -63.9071)
  arc A67 (21.7511, -63.9071) -> (22.1355, -63.7486) centre (21.9789, -63.9142) cw
  line L97 (47.0464, -57.0601) -> (25.8098, -57.0601)
  arc A68 (25.6618, -57.4183) -> (25.8098, -57.0601) centre (25.8098, -57.2698) cw
  line L98 (25.6618, -57.4183) -> (36.0691, -67.797)
  arc A69 (36.7874, -67.797) -> (36.0691, -67.797) centre (36.4282, -67.4369) cw
  line L99 (36.7874, -67.797) -> (47.1945, -57.4183)
  arc A70 (47.0464, -57.0601) -> (47.1945, -57.4183) centre (47.0464, -57.2698) cw
  line L100 (23.4063, -22.5552) -> (31.8695, -31.3349)
  arc A71 (31.8695, -31.3349) -> (31.8582, -32.054) centre (31.5024, -31.6888) cw
  line L101 (31.8582, -32.054) -> (22.8234, -40.8562)
  arc A72 (22.8234, -40.8562) -> (22.476, -40.7032) centre (22.6806, -40.7095) cw
  line L102 (22.476, -40.7032) -> (23.0385, -22.697)
  arc A73 (23.0385, -22.697) -> (23.4063, -22.5552) centre (23.2523, -22.7037) cw
  line L103 (49.4493, -22.5552) -> (40.9862, -31.3349)
  arc A74 (40.9975, -32.054) -> (40.9862, -31.3349) centre (41.3533, -31.6888) cw
  line L104 (40.9975, -32.054) -> (50.0325, -40.8562)
  arc A75 (50.38, -40.7032) -> (50.0325, -40.8562) centre (50.1754, -40.7095) cw
  line L105 (50.38, -40.7032) -> (49.8171, -22.697)
  arc A76 (49.4493, -22.5552) -> (49.8171, -22.697) centre (49.6033, -22.7037) cw
  line L106 (46.8177, -47.5501) -> (26.0383, -47.5501)
  arc A77 (26.0383, -47.5501) -> (25.8865, -47.1883) centre (26.0383, -47.3373) cw
  line L107 (25.8865, -47.1883) -> (36.0725, -36.817)
  arc A78 (36.0725, -36.817) -> (36.7833, -36.8169) centre (36.4279, -37.166) cw
  line L108 (36.7833, -36.8169) -> (46.9695, -47.1883)
  arc A79 (46.9695, -47.1883) -> (46.8177, -47.5501) centre (46.8177, -47.3373) cw
  line L109 (46.0554, -15.85) -> (26.8, -15.85)
  arc A80 (26.6349, -16.2245) -> (26.8, -15.85) centre (26.8, -16.0737) cw
  line L110 (26.6349, -16.2245) -> (36.0858, -26.5706)
  arc A81 (36.7699, -26.5706) -> (36.0858, -26.5706) centre (36.4278, -26.2581) cw
  line L111 (36.7699, -26.5706) -> (46.2205, -16.2245)
  arc A82 (46.0554, -15.85) -> (46.2205, -16.2245) centre (46.0554, -16.0737) cw
  line L112 (56.7216, -243.5837) -> (56.06, -222.4075)
  arc A83 (55.537, -221.9006) -> (56.06, -222.4075) centre (55.537, -222.4238) cw
  line L113 (55.537, -221.9006) -> (17.3225, -221.9006)
  arc A84 (16.7995, -222.4075) -> (17.3225, -221.9006) centre (17.3225, -222.4239) cw
  line L114 (16.7995, -222.4075) -> (16.1375, -243.5837)
  arc A85 (16.6289, -244.0906) -> (16.1375, -243.5837) centre (16.6289, -243.599) cw
  line L115 (16.6289, -244.0906) -> (56.2302, -244.0906)
  arc A86 (56.7216, -243.5837) -> (56.2302, -244.0906) centre (56.2302, -243.599) cw
  spline S0 degree 3 poles (36.4311, -34.1415) (35.0825, -34.1417) (33.989, -33.0487) (33.9885, -31.7001) knots 0 0 0 0 1 1 1 1
  spline S1 degree 3 poles (33.9885, -31.7001) (33.988, -30.3515) (35.0808, -29.2578) (36.4294, -29.2571) knots 0 0 0 0 1 1 1 1
  spline S2 degree 3 poles (36.4294, -29.2571) (37.778, -29.2564) (38.8719, -30.349) (38.8724, -31.6984) knots 0 0 0 0 1 1 1 1
  spline S3 degree 3 poles (38.8724, -31.6984) (38.8728, -33.0479) (37.7797, -34.1412) (36.4311, -34.1415) knots 0 0 0 0 1 1 1 1
extrude "Extrude3" add sketch "Sketch5" along normal blind 3.175 separate body contours L0 L1 A0 L2 A1 L3 L4 L5 A2 L6 A3 L7 L8 L9 A4 L10 A5 L11 L12 L13 A6 L14 A7 L15 L16 L17 A8 L18 A9 L19 L20 A10 L21 A11 L22 L23 A12 L24 L25 A13 L26 A14 L27 L28 L29 A15 L30 A16 L31 L32 A17 L33 A18 L34 A19 L35 L36 L37 A20 L38 A21 L39 L40 L41 A22 L42 A23 L43 L44 A24 L45 A25 L46 L47 A26 | L82 A53 L83 A54 L84 A55 | L88 A59 L89 A60 L90 A61 | L94 A65 L95 A66 L96 A67 makes body 3
move_body "Move3" bodies 3 to x (1, 0, 0) y (0, 1, 0) z (0, 0, 1) at (330.2, 0, 0)
copy_body "Body->Comp1" bodies 1 removing the originals makes body 4 in component "bottom"
copy_body "Body->Comp2" bodies 2 removing the originals makes body 5 in component "side"
copy_body "Body->Comp3" bodies 3 removing the originals makes body 6 in component "sidemirrored"
sketch "Sketch8" plane through (0, 0, 0) normal (0, 0, 1) x (1, 0, 0)
  line L0 (79.6139, -72.0608) -> (43.9249, -92.6658)
  arc A0 (43.9249, -92.6658) -> (38.4343, -92.6658) centre (41.1796, -87.9108) cw
  line L1 (38.4343, -92.6658) -> (2.7453, -72.0608)
  arc A1 (2.7453, -72.0608) -> (0, -67.3058) centre (5.4906, -67.3058) cw
  line L2 (0, -67.3058) -> (0, -26.0957)
  arc A2 (0, -26.0957) -> (2.7453, -21.3407) centre (5.4906, -26.0957) cw
  line L3 (2.7453, -21.3407) -> (38.4343, -0.7356)
  arc A3 (38.4343, -0.7356) -> (43.9249, -0.7356) centre (41.1796, -5.4906) cw
  line L4 (43.9249, -0.7356) -> (79.6139, -21.3407)
  arc A4 (79.6139, -21.3407) -> (82.3592, -26.0957) centre (76.8686, -26.0957) cw
  line L5 (82.3592, -26.0957) -> (82.3592, -67.3058)
  arc A5 (82.3592, -67.3058) -> (79.6139, -72.0608) centre (76.8686, -67.3058) cw
  line L6 (46.8442, -81.8721) -> (48.6934, -85.075)
  line L7 (48.6934, -85.075) -> (70.6558, -72.3949)
  line L8 (70.6558, -72.3949) -> (68.8066, -69.1921)
  line L9 (68.8066, -69.1921) -> (46.8442, -81.8721)
  line L10 (35.515, -81.8721) -> (33.6659, -85.075)
  line L11 (33.6659, -85.075) -> (11.7034, -72.3949)
  line L12 (11.7034, -72.3949) -> (13.5526, -69.1921)
  line L13 (13.5526, -69.1921) -> (35.515, -81.8721)
  line L14 (35.515, -11.5293) -> (33.6659, -8.3264)
  line L15 (33.6659, -8.3264) -> (11.7034, -21.0065)
  line L16 (11.7034, -21.0065) -> (13.5526, -24.2093)
  line L17 (13.5526, -24.2093) -> (35.515, -11.5293)
  line L18 (46.8442, -11.5293) -> (48.6934, -8.3264)
  line L19 (48.6934, -8.3264) -> (70.6558, -21.0065)
  line L20 (70.6558, -21.0065) -> (68.8066, -24.2093)
  line L21 (68.8066, -24.2093) -> (46.8442, -11.5293)
  line L22 (74.4712, -34.0207) -> (78.1696, -34.0207)
  line L23 (78.1696, -34.0207) -> (78.1696, -59.3807)
  line L24 (78.1696, -59.3807) -> (74.4712, -59.3807)
  line L25 (74.4712, -59.3807) -> (74.4712, -34.0207)
  line L26 (4.1896, -34.0207) -> (7.888, -34.0207)
  line L27 (7.888, -34.0207) -> (7.888, -59.3807)
  line L28 (7.888, -59.3807) -> (4.1896, -59.3807)
  line L29 (4.1896, -59.3807) -> (4.1896, -34.0207)
  line L30 (38.297, -77.4569) -> (38.297, -52.5581)
  arc A6 (37.5482, -52.1258) -> (38.297, -52.5581) centre (37.7978, -52.5581) cw
  line L31 (37.5482, -52.1258) -> (15.9853, -64.5752)
  arc A7 (15.9853, -65.4398) -> (15.9853, -64.5752) centre (16.2349, -65.0075) cw
  line L32 (15.9853, -65.4398) -> (37.5482, -77.8892)
  arc A8 (38.297, -77.4569) -> (37.5482, -77.8892) centre (37.7978, -77.4569) cw
  line L33 (44.0622, -77.4569) -> (44.0622, -52.5581)
  arc A9 (44.0622, -52.5581) -> (44.811, -52.1258) centre (44.5614, -52.5581) cw
  line L34 (44.811, -52.1258) -> (66.3739, -64.5752)
  arc A10 (66.3739, -64.5752) -> (66.3739, -65.4398) centre (66.1243, -65.0075) cw
  line L35 (66.3739, -65.4398) -> (44.811, -77.8892)
  arc A11 (44.811, -77.8892) -> (44.0622, -77.4569) centre (44.5614, -77.4569) cw
  line L36 (38.297, -15.9445) -> (38.297, -40.8433)
  arc A12 (38.297, -40.8433) -> (37.5482, -41.2756) centre (37.7978, -40.8433) cw
  line L37 (37.5482, -41.2756) -> (15.9853, -28.8263)
  arc A13 (15.9853, -28.8263) -> (15.9853, -27.9616) centre (16.2349, -28.3939) cw
  line L38 (15.9853, -27.9616) -> (37.5482, -15.5122)
  arc A14 (37.5482, -15.5122) -> (38.297, -15.9445) centre (37.7978, -15.9445) cw
  line L39 (47.6936, -46.2684) -> (69.2565, -33.819)
  arc A15 (69.2565, -33.819) -> (70.0053, -34.2513) centre (69.5061, -34.2513) cw
  line L40 (70.0053, -34.2513) -> (70.0053, -59.1501)
  arc A16 (70.0053, -59.1501) -> (69.2565, -59.5824) centre (69.5061, -59.1501) cw
  line L41 (69.2565, -59.5824) -> (47.6936, -47.133)
  arc A17 (47.6936, -47.133) -> (47.6936, -46.2684) centre (47.9432, -46.7007) cw
  line L42 (13.1027, -33.819) -> (34.6656, -46.2684)
  arc A18 (34.6656, -46.2684) -> (34.6656, -47.133) centre (34.416, -46.7007) cw
  line L43 (34.6656, -47.133) -> (13.1027, -59.5824)
  arc A19 (13.1027, -59.5824) -> (12.3539, -59.1501) centre (12.8531, -59.1501) cw
  line L44 (12.3539, -59.1501) -> (12.3539, -34.2513)
  arc A20 (12.3539, -34.2513) -> (13.1027, -33.819) centre (12.8531, -34.2513) cw
  line L45 (66.3739, -27.9616) -> (44.811, -15.5122)
  arc A21 (44.0622, -15.9445) -> (44.811, -15.5122) centre (44.5614, -15.9445) cw
  line L46 (44.0622, -15.9445) -> (44.0622, -40.8433)
  arc A22 (44.811, -41.2756) -> (44.0622, -40.8433) centre (44.5614, -40.8433) cw
  line L47 (44.811, -41.2756) -> (66.3739, -28.8263)
  arc A23 (66.3739, -27.9616) -> (66.3739, -28.8263) centre (66.1243, -28.3939) cw
  spline S0 degree 3 poles (41.1803, -49.1429) (39.8317, -49.1431) (38.7381, -48.0502) (38.7377, -46.7016) knots 0 0 0 0 1 1 1 1
  spline S1 degree 3 poles (38.7377, -46.7016) (38.7372, -45.353) (39.83, -44.2592) (41.1786, -44.2585) knots 0 0 0 0 1 1 1 1
  spline S2 degree 3 poles (41.1786, -44.2585) (42.5272, -44.2578) (43.6211, -45.3504) (43.6216, -46.6999) knots 0 0 0 0 1 1 1 1
  spline S3 degree 3 poles (43.6216, -46.6999) (43.622, -48.0493) (42.5289, -49.1427) (41.1803, -49.1429) knots 0 0 0 0 1 1 1 1
extrude "Extrude6" add sketch "Sketch8" along normal blind 3.175 separate body makes body 7
copy_body "Body->Comp6" bodies 7 removing the originals makes body 8 in component "Component"
component "bottom" placed x (1, 0, 0) y (0, 1, 0) z (0, 0, 1) at (0, 0, 0)
component "side" placed x (0.866026, 0.5, 0) y (-0.044013, 0.076232, 0.996118) z (0.498059, -0.862664, 0.088025) at (-56.2705, -243.1298, 255.8891)
component "sidemirrored" placed x (0, 1, 0) y (-0.088025, 0, 0.996118) z (0.996118, 0, 0.088025) at (201.0133, -441.8601, 255.8891)
component "side" placed x (-0.866026, 0.5, 0) y (-0.044012, -0.076232, 0.996118) z (0.498059, 0.862664, 0.088025) at (424.7712, -185.0609, 255.8891)
component "side" placed x (0, -1, 0) y (0.088025, 0, 0.996118) z (-0.996118, 0, 0.088025) at (133.9614, 202.4988, 255.8891)
component "sidemirrored" placed x (0.866026, -0.499999, 0) y (0.044012, 0.076232, 0.996118) z (-0.498058, -0.862664, 0.088025) at (-166.7863, 79.0494, 255.8891)
component "sidemirrored" placed x (-0.866026, -0.499999, 0) y (0.044012, -0.076232, 0.996118) z (-0.498059, 0.862664, 0.088025) at (468.2349, 137.1182, 255.8891)
component "Component" placed x (1, 0, 0) y (0, 1, 0) z (0, 0, 1) at (0, 0, 0)
